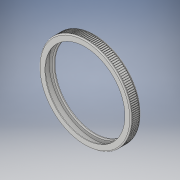
# Autodesk Inventor part: bepf_kolo_opona
Saved by Autodesk Inventor 2017 (Build 210142000, 142)
## iProperties
Created: 2016-11-23
Part Number: bepf_kolo_opona
Material: Ogólny
Document SubType Name: Modeling
Designer: gagato
Density: 1 g/cm^3
Appearance: Domyślna
Author: gagato
Autodesk Inventor part; units mm, degrees
ref_plane "XZ Plane" through (0, 0, 0) normal (0, 1, 0) x (-1, 0, 0)
ref_plane "XY Plane" through (0, 0, 0) normal (0, 0, 1) x (1, 0, 0)
sketch "Szkic1" plane through (0, 0, 0) normal (0, 0, 1) x (1, 0, 0)
  circle A0 centre (0, 0) radius 45
  circle A1 centre (0, 0) radius 39.25
  dimension "d0" = 90
  dimension "d1" = 78.5
  constraints: 2 centre point, 2 coincident
  measures "d0" diameter of A0
  measures "d1" diameter of A1
extrude "Wyciągnięcie proste1" add sketch "Szkic1" along normal mid plane 10
shell "Skorupa1" thickness 1.75 removed faces 2 at (38.8116, -5.8499, 3.3333) at (38.8116, -5.8499, -3.3333)
fillet "Zaokrąglenie1" radius 1 4 edges at (-39.25, 0, -3.25) (-39.25, 0, 3.25) (-45, 0, 5) (-45, 0, -5)
ref_plane "Płaszczyzna konstrukcyjna1" through (45, 0, 0) normal (1, 0, 0) x (0, 1, 0)
sketch "Szkic2" plane through (45, 0, 0) normal (1, 0, 0) x (0, 1, 0)
  line L0 (-0.75, -3.5) -> (-0.75, 3.5)
  line L1 (-0.75, 3.5) -> (0.75, 3.5)
  line L2 (0.75, 3.5) -> (0.75, -3.5)
  line L3 (0.75, -3.5) -> (-0.75, -3.5)
  line L4 (-0.75, -3.5) -> (0.75, 3.5) construction
  line L5 (-0.75, 3.5) -> (0.75, -3.5) construction
  point P0 (0, 0)
  dimension "d6" = 7
  dimension "d7" = 1.5
  constraints: 12 end point, 2 midpoint, 2 parallel, 1 perpendicular, 1 vertical
  measures "d6" distance of L0.start L0.end
  measures "d7" distance of L0.end L1.end
extrude "Wyciągnięcie proste2" cut sketch "Szkic2" against normal blind 0.5
pattern_circular "Szyk kołowy1" count 160 over 360 about axis through (0, 0, 0) along (0, 0, 1) of "Wyciągnięcie proste2"
